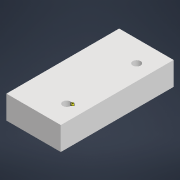
# Autodesk Inventor part: Part4
Saved by Autodesk Inventor 2022 (Build 260153000, 153)
## iProperties
Created: 2021-11-03
Part Number: Part4
Material: Generic
Document SubType Name: Modeling
Designer: 17185
Density: 1 g/cm^3
Appearance: Default
Author: 17185
Autodesk Inventor part; units mm, degrees
ref_plane "YZ Plane" through (0, 0, 0) normal (1, 0, 0) x (0, 1, 0)
ref_plane "XZ Plane" through (0, 0, 0) normal (0, 1, 0) x (-1, 0, 0)
ref_plane "XY Plane" through (0, 0, 0) normal (0, 0, 1) x (1, 0, 0)
sketch "Sketch1" plane through (0, 0, 0) normal (0, 1, 0) x (-1, 0, 0)
  line L0 (12.7, 46.0375) -> (-12.7, 46.0375)
  line L1 (-12.7, 46.0375) -> (-12.7, -46.0375)
  line L2 (-12.7, -46.0375) -> (12.7, -46.0375)
  line L3 (12.7, -46.0375) -> (12.7, 46.0375)
  line L4 (12.7, 46.0375) -> (-12.7, -46.0375) construction
  line L5 (-12.7, 46.0375) -> (12.7, -46.0375) construction
  circle A0 centre (0, -28.575) radius 3.175
  line L6 (7.8828, 28.575) -> (-7.8828, 28.575) construction
  line L7 (-7.8828, 28.575) -> (-7.8828, -28.575) construction
  line L8 (-7.8828, -28.575) -> (7.8828, -28.575) construction
  line L9 (7.8828, -28.575) -> (7.8828, 28.575) construction
  line L10 (7.8828, 28.575) -> (-7.8828, -28.575) construction
  line L11 (-7.8828, 28.575) -> (7.8828, -28.575) construction
  circle A1 centre (0, 28.575) radius 3.175
  line L12 (12.7, -46.0375) -> (31.75, -46.0375)
  line L13 (31.75, -46.0375) -> (31.75, 46.0375)
  line L14 (31.75, 46.0375) -> (12.7, 46.0375)
  line L15 (12.7, 46.0375) -> (12.7, -46.0375)
  point P0 (0, 0)
  point P1 (12.7, 46.0375)
  dimension "d0" = 92.075
  dimension "d1" = 25.4
  dimension "d4" = 6.35
  dimension "d5" = 6.35
  dimension "d6" = 28.575
  dimension "d11" = 19.05
  dimension "d12" = 92.075
  constraints: 32 end point, 6 midpoint, 6 parallel, 3 horizontal, 3 perpendicular, 2 centre point, 1 point on line
  measures "d0" distance of L0.end L1.end
  measures "d1" distance of L1.end L2.end
  measures "d4" diameter of A0
  measures "d5" diameter of A1
  measures "d6" distance from line of L8 point (0, 0)
  measures "d11" distance of L14.end L13.end
  measures "d12" distance of L12.end L13.end
extrude "Extrusion1" add sketch "Sketch1" along normal blind 19.05
body "Solid1"
